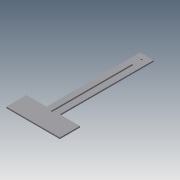
# Autodesk Inventor part: Part1
Saved by Autodesk Inventor 2015 (Build 190159000, 159)
## iProperties
Created: 2014-07-15
Part Number: Part1
Material: Generic
Document SubType Name: Modeling
Designer: shohei
Density: 1 g/cm^3
Appearance: Default
Mass: 1238.43 g
Surface Area: 2853.14 cm^2
Volume: 1238.43 cm^3
Author: shohei
Autodesk Inventor part; units mm, degrees
ref_plane "YZ Plane" through (0, 0, 0) normal (1, 0, 0) x (0, 1, 0)
ref_plane "XZ Plane" through (0, 0, 0) normal (0, 1, 0) x (-1, 0, 0)
ref_plane "XY Plane" through (0, 0, 0) normal (0, 0, 1) x (1, 0, 0)
sketch "Sketch1" plane through (0, 0, 0) normal (0, 0, 1) x (1, 0, 0)
  line L0 (-200, 0) -> (-200, 150)
  line L1 (-200, 150) -> (200, 150)
  line L2 (200, 150) -> (200, 0)
  line L3 (200, 0) -> (-200, 0)
  line L4 (50, 150) -> (-50, 150)
  line L5 (-50, 150) -> (-50, 850)
  line L6 (-50, 850) -> (50, 850)
  line L7 (50, 850) -> (50, 150)
  line L8 (0, -170) -> (0, 1020) projected
  line L9 (-280, 0) -> (280, 0) projected
  point P0 (0, 0)
  dimension "d7" = 700
  dimension "d11" = 50
  dimension "d12" = 50
  dimension "d13" = 200
  dimension "d14" = 200
  dimension "d15" = 150
  dimension "d17" = 200
  dimension "d18" = 200
  constraints: 16 end point, 3 parallel, 2 horizontal, 1 perpendicular, 1 point on line
  measures "d7" distance between parallel lines of L1 L6
  measures "d11" distance between parallel lines of L5 L8
  measures "d12" distance between parallel lines of L7 L8
  measures "d13" distance of L0.start point (0, 0)
  measures "d14" distance of L2.end point (0, 0)
  measures "d15" distance of L2.end L1.end
  measures "d17" distance from line of L8 L1.end
  measures "d18" distance from line of L8 L0.end
extrude "Extrusion2" add sketch "Sketch1" along normal blind 10
sketch "Sketch2" plane through (0, 0, 10) normal (0, 0, 1) x (1, 0, 0)
  line L0 (5, 140) -> (5, 740)
  line L1 (0, -170) -> (0, 1020) projected
  line L2 (-280, 0) -> (280, 0) projected
  arc A0 (0, 135) -> (5, 140) centre (0, 140) ccw
  line L3 (-5, 140) -> (-5, 740)
  arc A1 (-5, 140) -> (0, 135) centre (0, 140) ccw
  arc A2 (5, 740) -> (-5, 740) centre (0, 740) ccw
  line L4 (50, 850) -> (-50, 850) projected
  point P0 (0, 0)
  point P1 (0, 149.3301)
  dimension "d8" = 5
  dimension "d24" = 600
  dimension "d26" = 10
  dimension "d30" = 10
  dimension "d34" = 110
  constraints: 6 point on circle, 4 end point, 4 point on line, 3 centre point, 3 symmetric about line, 1 coincident, 1 vertical, 1 other
  measures "d8" distance between parallel lines of L0 L1
  measures "d24" distance of L0.end L0.start
  measures "d26" diameter of A0
  measures "d30" diameter of A2
  measures "d34" distance from line of L4 A2.centre
sketch "Sketch3" plane through (0, 0, 0) normal (0, 0, -1) x (-1, 0, 0)
  line L0 (0, -170) -> (0, 1020) projected
  line L1 (280, 0) -> (-280, 0) projected
  circle A0 centre (0, 810) radius 5
  line L2 (-50, 850) -> (50, 850) projected
  point P0 (0, 0)
  dimension "d19" = 10
  dimension "d27" = 40
  constraints: 1 centre point, 1 point on line
  measures "d19" diameter of A0
  measures "d27" distance from line of L2 A0.centre
extrude "Extrusion4" cut sketch "Sketch3" against normal through all
extrude "Extrusion6" cut sketch "Sketch2" against normal through all
body "Solid2"
